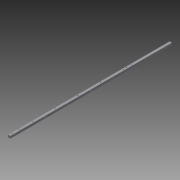
# Autodesk Inventor part: Plate Support
Saved by Autodesk Inventor 2015 SP1 (Build 190203100, 203)
## iProperties
Created: 2014-07-11
Part Number: Plate Support
Material: Generic
Document SubType Name: Modeling
Designer: I Rabey
Density: 1 g/cm^3
Appearance: Default
Author: I Rabey
Autodesk Inventor part; units mm, degrees
ref_plane "YZ Plane" through (0, 0, 0) normal (1, 0, 0) x (0, 1, 0)
ref_plane "XZ Plane" through (0, 0, 0) normal (0, 1, 0) x (-1, 0, 0)
ref_plane "XY Plane" through (0, 0, 0) normal (0, 0, 1) x (1, 0, 0)
sketch "Sketch1" plane through (0, 0, 0) normal (0, 1, 0) x (-1, 0, 0)
  line L0 (6.35, -451.5) -> (-6.35, -451.5)
  line L1 (-6.35, -451.5) -> (-6.35, 451.5)
  line L2 (-6.35, 451.5) -> (6.35, 451.5)
  line L3 (6.35, 451.5) -> (6.35, -451.5)
  line L4 (6.35, -451.5) -> (-6.35, 451.5) construction
  line L5 (-6.35, -451.5) -> (6.35, 451.5) construction
  point P0 (0, 0)
  dimension "d0" = 12.7
  dimension "d1" = 903
  constraints: 12 end point, 2 midpoint, 2 parallel, 1 horizontal, 1 perpendicular
  measures "d0" distance of L1.end L2.end
  measures "d1" distance of L0.end L1.end
extrude "Extrusion1" add sketch "Sketch1" along normal blind 12.7
sketch "Sketch2" plane through (0, 12.7, 0) normal (0, 1, 0) x (1, 0, 0)
  circle A0 centre (0, -434.99) radius 2.5
  line L0 (-6.35, -451.5) -> (6.35, -451.5) projected
  point P0 (0, 0)
  dimension "d4" = 5
  dimension "d5" = 16.51
  constraints: 1 centre point
  measures "d4" diameter of A0
  measures "d5" distance from line of A0.centre L0
sketch "Sketch3" plane through (0, 12.7, 0) normal (0, 1, 0) x (1, 0, 0)
  circle A0 centre (0, -396.89) radius 2.5
  line L0 (-6.35, -451.5) -> (6.35, -451.5) projected
  point P0 (0, 0)
  dimension "d6" = 5
  dimension "d7" = 54.61
  constraints: 1 centre point
  measures "d6" diameter of A0
  measures "d7" distance from line of L0 A0.centre
sketch "Sketch4" plane through (0, 12.7, 0) normal (0, 1, 0) x (1, 0, 0)
  circle A0 centre (0, -320.84) radius 2.5
  line L0 (-6.35, -451.5) -> (6.35, -451.5) projected
  point P0 (0, 0)
  dimension "d8" = 5
  dimension "d9" = 130.66
  constraints: 1 centre point
  measures "d8" diameter of A0
  measures "d9" distance from line of L0 A0.centre
sketch "Sketch5" plane through (0, 12.7, 0) normal (0, 1, 0) x (1, 0, 0)
  circle A0 centre (0, -193.84) radius 2.5
  line L0 (-6.35, -451.5) -> (6.35, -451.5) projected
  point P0 (0, 0)
  dimension "d10" = 5
  dimension "d11" = 257.66
  constraints: 1 centre point
  measures "d10" diameter of A0
  measures "d11" distance from line of L0 A0.centre
sketch "Sketch6" plane through (0, 12.7, 0) normal (0, 1, 0) x (1, 0, 0)
  circle A0 centre (0, -66.84) radius 2.5
  line L0 (-6.35, -451.5) -> (6.35, -451.5) projected
  point P0 (0, 0)
  dimension "d12" = 5
  dimension "d13" = 384.66
  constraints: 1 centre point
  measures "d12" diameter of A0
  measures "d13" distance from line of L0 A0.centre
sketch "Sketch7" plane through (0, 12.7, 0) normal (0, 1, 0) x (1, 0, 0)
  circle A0 centre (0, 60.16) radius 2.5
  line L0 (-6.35, -451.5) -> (6.35, -451.5) projected
  point P0 (0, 0)
  dimension "d14" = 5
  dimension "d15" = 511.66
  constraints: 1 centre point
  measures "d14" diameter of A0
  measures "d15" distance from line of L0 A0.centre
sketch "Sketch8" plane through (0, 12.7, 0) normal (0, 1, 0) x (1, 0, 0)
  circle A0 centre (0, 187.16) radius 2.5
  line L0 (-6.35, -451.5) -> (6.35, -451.5) projected
  point P0 (0, 0)
  dimension "d16" = 5
  dimension "d17" = 638.66
  constraints: 1 centre point
  measures "d16" diameter of A0
  measures "d17" distance from line of L0 A0.centre
sketch "Sketch9" plane through (0, 12.7, 0) normal (0, 1, 0) x (1, 0, 0)
  circle A0 centre (0, 205.24) radius 2.5
  line L0 (-6.35, -451.5) -> (6.35, -451.5) projected
  point P0 (0, 0)
  dimension "d18" = 5
  dimension "d19" = 656.74
  constraints: 1 centre point
  measures "d18" diameter of A0
  measures "d19" distance from line of L0 A0.centre
sketch "Sketch10" plane through (0, 12.7, 0) normal (0, 1, 0) x (1, 0, 0)
  circle A0 centre (0, 230.64) radius 2.5
  line L0 (-6.35, -451.5) -> (6.35, -451.5) projected
  point P0 (0, 0)
  dimension "d20" = 5
  dimension "d21" = 682.14
  constraints: 1 centre point
  measures "d20" diameter of A0
  measures "d21" distance from line of L0 A0.centre
hole "Hole1" at (0, 12.7, 434.99) direction (0, -1, 0) diameter 5 end through all
hole "Hole2" at (0, 12.7, 396.89) direction (0, -1, 0) diameter 5 end through all
hole "Hole3" at (0, 12.7, 320.84) direction (0, -1, 0) diameter 5 end through all
hole "Hole4" at (0, 12.7, 193.84) direction (0, -1, 0) diameter 5 end through all
hole "Hole5" at (0, 12.7, 66.84) direction (0, -1, 0) diameter 5 end through all
hole "Hole6" at (0, 12.7, -60.16) direction (0, -1, 0) diameter 5 end through all
hole "Hole7" at (0, 12.7, -187.16) direction (0, -1, 0) diameter 5 end through all
hole "Hole8" at (0, 12.7, -205.24) direction (0, -1, 0) diameter 5 end through all
hole "Hole9" at (0, 12.7, -230.64) direction (0, -1, 0) diameter 5 end through all
sketch "Sketch11" plane through (6.35, 0, -451.5) normal (0, 0, -1) x (-1, 0, 0)
  circle A0 centre (6.35, 6.35) radius 1.5
  line L0 (0, 0) -> (0, 12.7) projected
  point P0 (6.35, 0)
  dimension "d85" = 3
  dimension "d86" = 6.35
  dimension "d87" = 6.35
  constraints: 1 centre point
  measures "d85" diameter of A0
  measures "d86" distance from line of A0.centre L0
  measures "d87" distance of point (6.35, 0) A0.centre
hole "Hole10" at (0, 6.35, -451.5) direction (0, 0, 1) diameter 3 depth 8 tip angle 118
thread "Thread1" size "M3x0.5" class "6H" standard "ANSI Metric M Profile" full length
sketch "Sketch12" plane through (6.35, 0, 451.5) normal (1, 0, 0) x (0, 0, -1)
  circle A0 centre (194.16, 7.3065) radius 2.5
  line L0 (0, 0) -> (0, 12.7) projected
  point P0 (451.5, 0)
  dimension "d97" = 5
  dimension "d98" = 194.16
  constraints: 1 centre point
  measures "d97" diameter of A0
  measures "d98" distance from line of L0 A0.centre
sketch "Sketch13" plane through (6.35, 0, 451.5) normal (1, 0, 0) x (0, 0, -1)
  circle A0 centre (321.16, 7.3065) radius 2.5
  line L0 (0, 0) -> (0, 12.7) projected
  point P0 (451.5, 0)
  dimension "d99" = 5
  dimension "d100" = 321.16
  constraints: 1 centre point
  measures "d99" diameter of A0
  measures "d100" distance from line of L0 A0.centre
sketch "Sketch14" plane through (6.35, 0, 451.5) normal (1, 0, 0) x (0, 0, -1)
  circle A0 centre (448.16, 7.3065) radius 2.5
  line L0 (0, 0) -> (0, 12.7) projected
  point P0 (451.5, 0)
  dimension "d101" = 5
  dimension "d102" = 448.16
  constraints: 1 centre point
  measures "d101" diameter of A0
  measures "d102" distance from line of L0 A0.centre
sketch "Sketch15" plane through (6.35, 0, 451.5) normal (1, 0, 0) x (0, 0, -1)
  circle A0 centre (575.16, 7.3065) radius 2.5
  line L0 (0, 0) -> (0, 12.7) projected
  point P0 (451.5, 0)
  dimension "d103" = 5
  dimension "d104" = 575.16
  constraints: 1 centre point
  measures "d103" diameter of A0
  measures "d104" distance from line of L0 A0.centre
hole "Hole11" at (6.35, 7.3065, 257.34) direction (-1, 0, 0) diameter 5 end through all
hole "Hole12" at (6.35, 7.3065, 130.34) direction (-1, 0, 0) diameter 5 end through all
hole "Hole13" at (6.35, 7.3065, 3.34) direction (-1, 0, 0) diameter 5 end through all
hole "Hole14" at (6.35, 7.3065, -123.66) direction (-1, 0, 0) diameter 5 end through all
body "Solid1"
